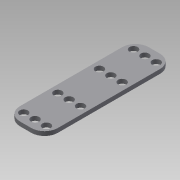
# Autodesk Inventor part: SideToSide
Saved by Autodesk Inventor 2014 (Build 180170000, 170)
## iProperties
Created: 2014-03-07
Part Number: SideToSide
Material: Générique
Document SubType Name: Modeling
Designer: Grégoire
Density: 1 g/cm^3
Appearance: Par défaut
Author: Grégoire
Autodesk Inventor part; units mm, degrees
ref_plane "YZ Plane" through (0, 0, 0) normal (1, 0, 0) x (0, 1, 0)
ref_plane "XZ Plane" through (0, 0, 0) normal (0, 1, 0) x (-1, 0, 0)
ref_plane "XY Plane" through (0, 0, 0) normal (0, 0, 1) x (1, 0, 0)
sketch "Esquisse12" plane through (0, 0, 0) normal (0, 0, 1) x (1, 0, 0)
  line L0 (0, 0) -> (20, 0)
  line L1 (20, 0) -> (20, 34)
  line L2 (20, 34) -> (0, 34)
  line L3 (0, 34) -> (0, 0)
  line L4 (10, 34) -> (10, 0) construction
  circle A0 centre (10, 5) radius 2.15
  line L5 (10, 5) -> (20, 5) construction
  circle A1 centre (16, 5) radius 2.15
  circle A2 centre (4, 5) radius 2.15
  circle A3 centre (10, 5) radius 2.15
  circle A4 centre (10, 23) radius 2.15
  circle A5 centre (16, 23) radius 2.15
  circle A6 centre (4, 23) radius 2.15
  dimension "d133" = 20
  dimension "d134" = 5
  dimension "d135" = 4.3
  dimension "d138" = 6
  dimension "d141" = 6
  dimension "d148" = 18
  dimension "d153" = 11
  constraints: 12 end point, 7 centre point, 3 horizontal, 2 midpoint, 2 parallel, 2 perpendicular, 2 point on line, 1 vertical, 12 other
  measures "d133" distance of L0.start L0.end
  measures "d134" distance from line of L0 L5.start
  measures "d135" diameter of A0
  measures "d138" distance of L5.start A1.centre
  measures "d141" distance of L5.start A2.centre
  measures "d148" distance of A2.centre A6.centre
  measures "d153" distance from line of A4.centre L2
extrude "Extrusion13" add sketch "Esquisse12" along normal blind 2.2
fillet "Congé8" radius 7 2 edges at (20, 0, 1.1) (0, 0, 1.1)
mirror "Symétrie3" about plane through (20, 34, 0) normal (0, 1, 0)
equation "\"d135\" = Holes"
equation "\"d154\" = Depth"
equation "\"d156\" = Rounding"
equation "\"Depth\" = 2.2"
equation "\"Holes\" = 4.3"
equation "\"Height\" = 0"
equation "\"Rounding\" = 7"
